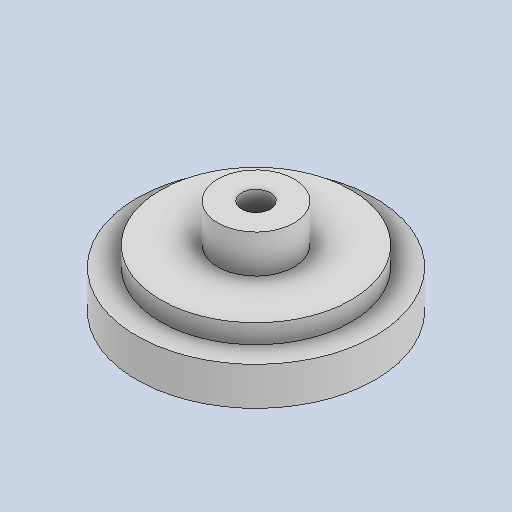
# Autodesk Inventor part: NEWWHEELS
Saved by Autodesk Inventor 2025 (Build 290162010, 162A)
## iProperties
Created: 2024-08-26
Part Number: NEWWHEELS
Material: Generic
Document SubType Name: Modeling
Designer: darkb
Density: 1 g/cm^3
Appearance: Default
Author: darkb
Autodesk Inventor part; units mm, degrees
ref_plane "YZ Plane" through (0, 0, 0) normal (1, 0, 0) x (0, 1, 0)
ref_plane "XZ Plane" through (0, 0, 0) normal (0, 1, 0) x (-1, 0, 0)
ref_plane "XY Plane" through (0, 0, 0) normal (0, 0, 1) x (1, 0, 0)
sketch "Sketch1" plane through (0, 0, 0) normal (0, 1, 0) x (-1, 0, 0)
  circle A0 centre (0, 0) radius 12.7
  dimension "d1" = 25.4
  constraints: 1 centre point
  measures "d1" diameter of A0
extrude "Extrusion3" add sketch "Sketch1" along normal blind 5.08
sketch "Sketch3" plane through (0, 0, 0) normal (0, -1, 0) x (1, 0, 0)
  circle A0 centre (0, 0) radius 0.4685
  constraints: 1 centre point, 1 coincident
hole "Hole1" at (0, 0, 0) direction (0, 1, 0) diameter 5.08 end through all counterbore diameter 38.1 counterbore depth 2.54
sketch "Sketch4" plane through (0, 2.54, 0) normal (0, -1, 0) x (1, 0, 0)
  circle A0 centre (0, 0) radius 11.9796
  circle A1 centre (0, 0) radius 19.05
  circle A2 centre (0, 0) radius 15.8934
  constraints: 3 centre point, 3 coincident
extrude "Extrusion4" add sketch "Sketch4" along normal blind 5.08 contours A2
sketch "Sketch5" plane through (0, 5.08, 0) normal (0, 1, 0) x (1, 0, 0)
  point P0 (0, 0)
sketch "Sketch6" plane through (0, 5.08, 0) normal (0, 1, 0) x (1, 0, 0)
  circle A0 centre (0, 0) radius 5.08
  dimension "d19" = 10.16
  constraints: 1 centre point, 1 coincident
  measures "d19" diameter of A0
sketch "Sketch7" plane through (0, 5.08, 0) normal (0, 1, 0) x (1, 0, 0)
  circle A0 centre (0, 0) radius 1.905
  dimension "d24" = 3.81
  constraints: 1 centre point, 1 coincident
  measures "d24" diameter of A0
extrude "Extrusion5" add sketch "Sketch6" along normal blind 5.08
extrude "Extrusion6" cut sketch "Sketch7" along normal blind 5.08
body "Solid2"
